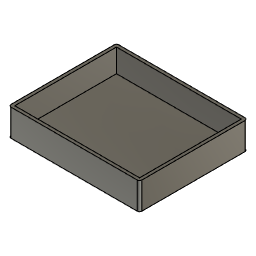
Potinho de agua v1 (Autodesk Fusion 360 design; units mm, degrees)
Autodesk Fusion 360 part; units mm, degrees
sketch "Esboço1" plane through (0, 0, 0) normal (0, 0, 1) x (1, 0, 0)
  line L0 (85, -70) -> (-85, -70)
  line L1 (-85, -70) -> (-85, 70)
  line L2 (-85, 70) -> (85, 70)
  line L3 (85, 70) -> (85, -70)
  line L4 (85, -70) -> (-85, 70) construction
  line L5 (-85, -70) -> (85, 70) construction
  dimension "d1" = 170
  dimension "d2" = 140
  constraint horizontal L0
  constraint perpendicular L0 L1
  constraint parallel L0 L2
  constraint parallel L1 L3
  constraint coincident L4 origin
  constraint coincident L5 origin
  measures "d1" distance of L1.end L2.end
  measures "d2" distance of L0.end L1.end
extrude "Extrusão1" add sketch "Esboço1" along normal blind 35
sketch "Esboço2" plane through (0, 0, 35) normal (0, 0, 1) x (-1, 0, 0)
  line L0 (-85, -70) -> (85, -70)
  line L1 (85, -70) -> (85, 70)
  line L2 (85, 70) -> (-85, 70)
  line L3 (-85, 70) -> (-85, -70)
  line L4 (-81, 66) -> (81, 66)
  line L5 (81, 66) -> (81, -66)
  line L6 (81, -66) -> (-81, -66)
  line L7 (-81, -66) -> (-81, 66)
  line L8 (-81, 66) -> (81, -66) construction
  line L9 (81, 66) -> (-81, -66) construction
  dimension "d5" = 162
  dimension "d6" = 132
  constraint horizontal L4
  constraint perpendicular L4 L5
  constraint parallel L4 L6
  constraint parallel L5 L7
  constraint coincident L8 origin
  constraint coincident L9 origin
  measures "d5" distance of L5.end L6.end
  measures "d6" distance of L4.end L5.end
extrude "Extrusão2" cut sketch "Esboço2" against normal blind 30 contours L4 L5 L6 L7
fillet "Arredondamento1" radius 3 4 edges at (-85, 70, 17.5) (-85, -70, 17.5) (85, -70, 17.5) (85, 70, 17.5)
